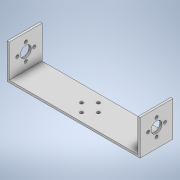
# Autodesk Inventor part: Rotate Brace
Saved by Autodesk Inventor 2020 (Build 240168000, 168)
## iProperties
Created: 2020-01-19
Part Number: Rotate Brace
Material: Generic
Document SubType Name: Modeling
Designer: tdmp4
Density: 1 g/cm^3
Appearance: Default
Author: tdmp4
Autodesk Inventor part; units mm, degrees
ref_plane "YZ Plane" through (0, 0, 0) normal (1, 0, 0) x (0, 1, 0)
ref_plane "XZ Plane" through (0, 0, 0) normal (0, 1, 0) x (-1, 0, 0)
ref_plane "XY Plane" through (0, 0, 0) normal (0, 0, 1) x (1, 0, 0)
sketch "Sketch1" plane through (0, 0, 0) normal (0, 1, 0) x (-1, 0, 0)
  line L0 (0, 0) -> (154.0002, 0)
  line L1 (154.0002, 0) -> (154.0002, -38.1)
  line L2 (154.0002, -38.1) -> (0, -38.1)
  line L3 (0, -38.1) -> (0, 0)
  dimension "d0" = 154.0002
  dimension "d1" = 38.1
  constraints: 8 end point, 2 parallel, 1 horizontal, 1 perpendicular
  measures "d0" distance of L1.end L2.end
  measures "d1" distance of L2.end L0.start
extrude "Extrusion1" add sketch "Sketch1" along normal blind 2.54
sketch "Sketch3" plane through (0, 0, 0) normal (1, 0, 0) x (0, 0, -1)
  circle A0 centre (19.05, 31.369) radius 1.7907
  circle A1 centre (28.829, 21.59) radius 1.7907
  circle A2 centre (19.05, 11.811) radius 1.7907
  circle A3 centre (9.271, 21.59) radius 1.7907
  circle A4 centre (19.05, 21.59) radius 6.35
  point P0 (0, 0)
  dimension "d12" = 12.7
  constraints: 5 centre point
  measures "d12" diameter of A4
sketch "Sketch4" plane through (0, 2.54, 0) normal (0, 1, 0) x (1, 0, 0)
  line L0 (0, 38.1) -> (-154.0002, 38.1) projected
  line L1 (0, 0) -> (-2.451, 0)
  line L2 (-2.451, 0) -> (-2.451, 38.1)
  line L3 (-2.451, 38.1) -> (0, 38.1)
  line L4 (0, 38.1) -> (0, 0)
  line L5 (-154.0002, 38.1) -> (-154.0002, 0) projected
  line L6 (-154.0002, 0) -> (-151.4602, 0)
  line L7 (-151.4602, 0) -> (-151.4602, 38.1)
  line L8 (-151.4602, 38.1) -> (-154.0002, 38.1)
  line L9 (-154.0002, 38.1) -> (-154.0002, 0)
  point P0 (0, 38.1)
  point P1 (-151.4602, 38.1)
  dimension "d17" = 2.54
  constraints: 16 end point, 4 parallel, 2 horizontal, 2 perpendicular, 2 point on line
  measures "d17" distance of L5.end L6.end
extrude "Extrusion3" add sketch "Sketch4" along normal blind 38.1
extrude "Extrusion4" cut sketch "Sketch3" against normal blind 203.2
sketch "Sketch5" plane through (0, 2.54, 0) normal (0, 1, 0) x (1, 0, 0)
  line L0 (0, 20.8407) -> (0, 17.2593) projected
  line L1 (-154.0002, 38.1) -> (-154.0002, 0) projected
  line L2 (-77.0001, 38.1) -> (-77.0001, 0)
  line L3 (-77.0001, 19.05) -> (-154.0002, 19.05)
  circle A0 centre (-77.0001, 19.05) radius 9.779
  circle A1 centre (-86.7791, 19.05) radius 1.7907
  circle A2 centre (-77.0001, 9.271) radius 1.7907
  circle A3 centre (-77.0001, 28.829) radius 1.7907
  circle A4 centre (-67.2211, 19.05) radius 1.7907
  point P0 (0, 0)
  dimension "d18" = 19.558
  dimension "d19" = 3.5814
  dimension "d20" = 3.5814
  dimension "d21" = 3.5814
  dimension "d22" = 3.5814
  constraints: 5 centre point, 4 end point, 4 point on circle, 3 point on line, 2 midpoint, 1 coincident, 1 vertical
  measures "d18" diameter of A0
  measures "d19" diameter of A1
  measures "d20" diameter of A2
  measures "d21" diameter of A3
  measures "d22" diameter of A4
extrude "Extrusion5" cut sketch "Sketch5" against normal blind 203.2 contours A3 A0 L2 | L2 A0 A3 | A0 A3 L2 | L2 A3 A0 | A1 L3 A0 | A0 L3 A1 | A4 A0 | A0 A4 | A0 A1 L3 | L3 A1 A0 | A2 A0 L2 | L2 A0 A2 | A0 A2 L2 | L2 A2 A0
body "Solid1"
